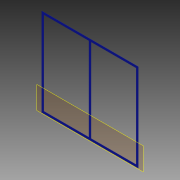
# Autodesk Inventor part: Tape
Saved by Autodesk Inventor 2013 (Build 170138000, 138)
## iProperties
Created: 2013-01-04
Part Number: Tape
Material: Polycarbonate, Clear
Document SubType Name: Modeling
Designer: Phillip
Density: 1 g/cm^3
Author: Phillip
Autodesk Inventor part; units mm, degrees
ref_plane "YZ Plane" through (0, 0, 0) normal (1, 0, 0) x (0, 1, 0)
ref_plane "XZ Plane" through (0, 0, 0) normal (0, 1, 0) x (-1, 0, 0)
ref_plane "XY Plane" through (0, 0, 0) normal (0, 0, 1) x (1, 0, 0)
ref_plane "Work Plane2" through (546.1, -990.6, 0) normal (0, 0, 1) x (1, 0, 0)
sketch "Sketch2" plane through (546.1, -990.6, 0) normal (0, 0, 1) x (1, 0, 0)
  line L0 (-1092.2, -238.125) -> (1092.2, -238.125)
  line L1 (1092.2, -238.125) -> (1092.2, 1749.425)
  line L2 (1092.2, 1749.425) -> (-1092.2, 1749.425)
  line L3 (-1092.2, 1749.425) -> (-1092.2, -238.125)
  line L4 (1041.4, 1698.625) -> (1041.4, -187.325)
  line L5 (-1041.4, -187.325) -> (-1041.4, 1698.625)
  line L6 (0, 231.775) -> (0, 1749.425) projected
  line L7 (-25.4, 1698.625) -> (-25.4, -187.325)
  line L8 (25.4, -187.325) -> (25.4, 1698.625)
  line L9 (-1041.4, 1698.625) -> (-25.4, 1698.625)
  line L10 (25.4, 1698.625) -> (1041.4, 1698.625)
  line L11 (1041.4, -187.325) -> (25.4, -187.325)
  line L12 (-25.4, -187.325) -> (-1041.4, -187.325)
  point P0 (-546.1, 990.6)
  point P1 (1092.2, -238.125)
  dimension "d12" = 50.8
  dimension "d13" = 25.4
  constraints: 24 end point, 7 parallel, 7 perpendicular, 1 horizontal, 4 other
  measures "d12" distance between parallel lines of L8 L7
  measures "d13" distance between parallel lines of L6 L7
extrude "Extrusion2" add sketch "Sketch2" along normal blind 2.54
body "Solid2"
